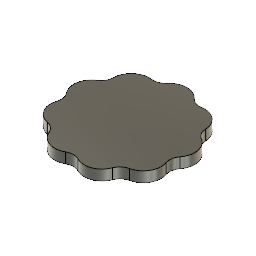
3.7 sweep (Autodesk Fusion 360 design; units mm, degrees)
Autodesk Fusion 360 part; units mm, degrees
sketch "Sketch3" plane through (0, 0, 0) normal (0, 0, 1) x (1, 0, 0)
  arc A0 (12.1503, 52.1262) -> (-13.4843, 51.7971) centre (-0.5229, 40.7362) ccw
  arc A1 (42.8137, 32.1209) -> (22.965, 48.3464) centre (25.7842, 31.5419) ccw
  arc A2 (53.4441, -2.9141) -> (48.6687, 22.2739) centre (40.0266, 7.5887) ccw
  arc A3 (39.0674, -36.5855) -> (51.5997, -14.2208) centre (35.5401, -19.9153) ccw
  arc A4 (6.4107, -53.1382) -> (30.3867, -44.0615) centre (14.424, -38.1007) ccw
  arc A5 (-29.2457, -44.8269) -> (-5.0446, -53.2853) centre (-13.4412, -38.4584) ccw
  arc A6 (-51.2177, -15.5406) -> (-38.1155, -37.5763) centre (-35.0172, -20.821) ccw
  arc A7 (-24.1984, 47.741) -> (-43.6241, 31.0114) centre (-26.5853, 30.8696) ccw
  arc A8 (-49.2244, 21.0173) -> (-53.3517, -4.2849) centre (-40.2082, 6.5588) ccw
  arc A9 (-49.2244, 21.0173) -> (-43.6241, 31.0114) centre (-55.5183, 31.1103) ccw
  arc A10 (-24.1984, 47.741) -> (-13.4843, 51.7971) centre (-22.5322, 59.5183) ccw
  arc A11 (12.1503, 52.1262) -> (22.965, 48.3464) centre (20.997, 60.0771) ccw
  arc A12 (42.8137, 32.1209) -> (48.6687, 22.2739) centre (54.7014, 32.5251) ccw
  arc A13 (53.4441, -2.9141) -> (51.5997, -14.2208) centre (62.8105, -10.2457) ccw
  arc A14 (39.0674, -36.5855) -> (30.3867, -44.0615) centre (41.5298, -48.2225) ccw
  arc A15 (6.4107, -53.1382) -> (-5.0446, -53.2853) centre (0.8168, -63.6354) ccw
  arc A16 (-29.2457, -44.8269) -> (-38.1155, -37.5763) centre (-40.2783, -49.2726) ccw
  arc A17 (-51.2177, -15.5406) -> (-53.3517, -4.2849) centre (-62.5268, -11.8546) ccw
  dimension "d14" = 11.8946
  measures "d14" radius of A9
extrude "Extrude1" add sketch "Sketch3" along normal blind 10
